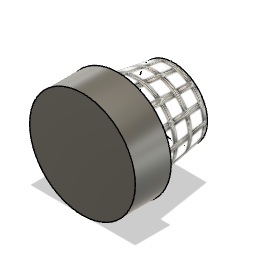
Rough Idea of PCB footprint v27 (Autodesk Fusion 360 archive; units mm, degrees)
design "MQ-4"
Autodesk Fusion 360 part; units mm, degrees
sketch "Sketch1" plane through (0, 0, 0) normal (0, 0, 1) x (1, 0, 0)
  circle A0 centre (0, 0) radius 6.15
  dimension "d1" = 12.3
  constraint coincident A0.centre origin
  measures "d1" diameter of A0
ref_plane "WorkPlane1" through (0, 0, 10) normal (0, 0, 1) x (1, 0, 0)
sketch "Sketch2" plane through (0, 0, 10) normal (0, 0, 1) x (1, 0, 0)
  circle A0 centre (0, 0) radius 7.75
  dimension "d3" = 15.5
  constraint coincident A0.centre origin
  measures "d3" diameter of A0
loft "Loft1" add profiles "Sketch2", "Sketch1" section 1 section 2
sketch "Sketch3" plane through (0, 0, 10) normal (0, 0, 1) x (1, 0, 0)
  circle A0 centre (0, 0) radius 7.75
  circle A1 centre (0, 0) radius 9.575
  dimension "d4" = 19.15
  constraint coincident A0.centre A1.centre
  measures "d4" diameter of A1
extrude "Extrude1" add sketch "Sketch3" along normal blind 6.5 contours A0 | A1
sketch "Sketch4" plane through (0, 0, 16.5) normal (0, 0, 1) x (1, 0, 0)
  circle A0 centre (0, 0) radius 9.575
  circle A1 centre (0, 0) radius 5.25 construction
  line L0 (0, 5.25) -> (0, -5.25) construction
  circle A2 centre (0, 5.25) radius 0.5
  circle A3 centre (-3.7123, 3.7123) radius 0.5
  circle A4 centre (-3.7123, -3.7123) radius 0.5
  circle A5 centre (0, -5.25) radius 0.5
  circle A6 centre (3.7123, -3.7123) radius 0.5
  circle A7 centre (3.7123, 3.7123) radius 0.5
  dimension "d7" = 10.5
  dimension "d8" = 1
  dimension "d10" = 360
  constraint coincident A0.centre A1.centre
  constraint coincident A1 L0.start
  constraint coincident A1 L0.end
  constraint vertical L0
  constraint coincident L0.start A2.centre
  measures "d7" diameter of A1
  measures "d8" diameter of A2

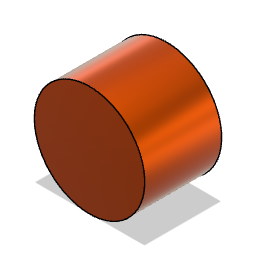
design "Gas sensor General volume"
Autodesk Fusion 360 part; units mm, degrees
sketch "Sketch1" plane through (0, 0, 0) normal (0, 0, 1) x (1, 0, 0)
  circle A0 centre (0, 0) radius 8.25
  dimension "d1" = 16.5
  constraint coincident A0.centre origin
  measures "d1" diameter of A0
extrude "Extrude1" add sketch "Sketch1" along normal blind 11.5
